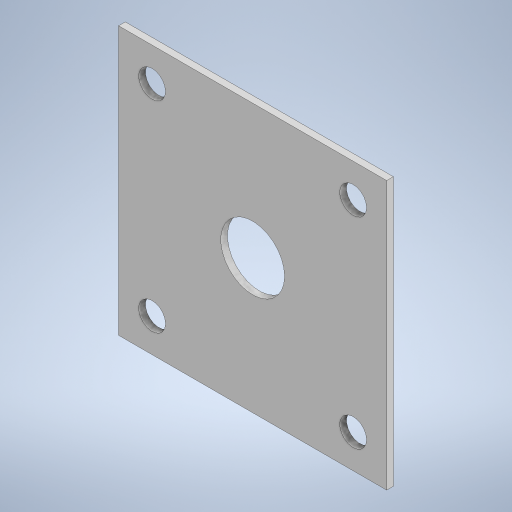
# Autodesk Inventor part: plate
Saved by Autodesk Inventor 2023 (Build 270158000, 158)
## iProperties
Created: 2022-09-29
Part Number: plate
Material: Generic
Document SubType Name: Sheet Metal
Designer: earls
Density: 1 g/cm^3
Sheet Metal Rule: Default_mm
Appearance: Default
Author: earls
Autodesk Inventor part; units mm, degrees
ref_plane "YZ Plane" through (0, 0, 0) normal (1, 0, 0) x (0, 1, 0)
ref_plane "XZ Plane" through (0, 0, 0) normal (0, 1, 0) x (-1, 0, 0)
ref_plane "XY Plane" through (0, 0, 0) normal (0, 0, 1) x (1, 0, 0)
sketch "Sketch1" plane through (0, 0, 0) normal (0, 0, 1) x (1, 0, 0)
  line L0 (-10.9665, 63.5108) -> (69.0335, 63.5108)
  line L1 (69.0335, 63.5108) -> (69.0335, -16.4892)
  line L2 (69.0335, -16.4892) -> (-10.9665, -16.4892)
  line L3 (-10.9665, -16.4892) -> (-10.9665, 63.5108)
  circle A0 centre (-0.9665, 53.5108) radius 4
  line L4 (29.0335, 63.5108) -> (29.0335, 23.5108)
  line L5 (-10.9665, 23.5108) -> (29.0335, 23.5108)
  circle A1 centre (59.0335, 53.5108) radius 4
  circle A2 centre (-0.9665, -6.4892) radius 4
  circle A3 centre (59.0335, -6.4892) radius 4
  circle A4 centre (29.0335, 23.5108) radius 9.525
  point P0 (0, 0)
  dimension "d0" = 80
  dimension "d1" = 80
  dimension "d2" = 8
  dimension "d3" = 10
  dimension "d4" = 10
  dimension "d7" = 19.05
  constraints: 12 end point, 5 centre point, 3 symmetric about line, 2 horizontal, 2 midpoint, 2 parallel, 1 coincident, 1 perpendicular, 1 vertical, 3 other
  measures "d0" distance of L0.start L0.end
  measures "d1" distance of L0.end L1.end
  measures "d2" diameter of A0
  measures "d3" distance from line of A0.centre L0
  measures "d4" distance from line of A0.centre L3
  measures "d7" diameter of A4
extrude "Plate1" add sketch "Sketch1" along normal mid plane 2
extrude "Cut1" cut sketch "Sketch1" against normal mid plane 2 contours A4 L5 L4 | L4 L5 A4
equation "\"d8\" = Thickness"
equation "\"d5\" = Thickness"
equation "\"BendRadius\" = Thickness"
equation "\"BendReliefWidth\" = Thickness"
equation "\"BendReliefDepth\" = 0.5 * Thickness"
equation "\"CornerReliefSize\" = 4 * Thickness"
equation "\"MinimumRemnant\" = 2 * Thickness"
equation "\"TransitionRadius\" = BendRadius"
equation "\"JacobiRadiusSize\" = BendRadius"
equation "\"GapSize\" = Thickness"
equation "\"Thickness\" = 2"
body "Solid1"
